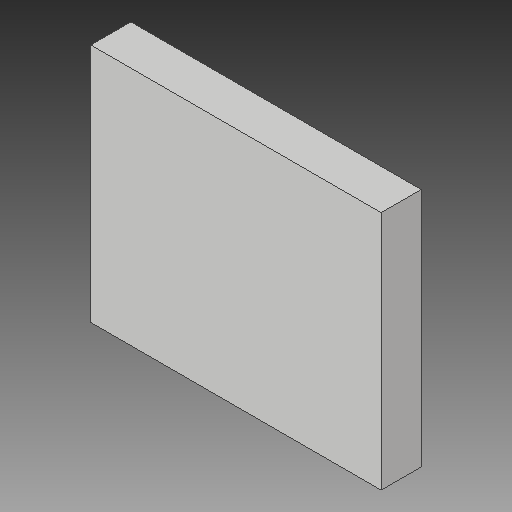
# Autodesk Inventor part: Ball screw nut and apron join
Saved by Autodesk Inventor 2018 (Build 220112000, 112)
## iProperties
Created: 2017-06-13
Part Number: Ball screw nut and apron join
Material: Generic
Document SubType Name: Modeling
Designer: m228540
Density: 1 g/cm^3
Appearance: Default
Author: m228540
Autodesk Inventor part; units mm, degrees
ref_plane "YZ Plane" through (0, 0, 0) normal (1, 0, 0) x (0, 1, 0)
ref_plane "XZ Plane" through (0, 0, 0) normal (0, 1, 0) x (-1, 0, 0)
ref_plane "XY Plane" through (0, 0, 0) normal (0, 0, 1) x (1, 0, 0)
sketch "Sketch1" plane through (0, 0, 0) normal (0, 0, 1) x (1, 0, 0)
  line L0 (-25.4985, 25.2291) -> (32.5015, 25.2291)
  line L1 (32.5015, 25.2291) -> (32.5015, -22.7709)
  line L2 (32.5015, -22.7709) -> (-25.4985, -22.7709)
  line L3 (-25.4985, -22.7709) -> (-25.4985, 25.2291)
  point P0 (0, 0)
  dimension "d0" = 58
  dimension "d1" = 48
  constraints: 8 end point, 2 parallel, 1 horizontal, 1 perpendicular
  measures "d0" distance of L0.start L0.end
  measures "d1" distance of L2.end L0.start
extrude "Extrusion1" add sketch "Sketch1" along normal blind 8
body "Solid1"
